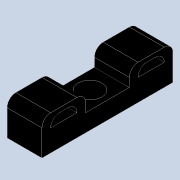
# Autodesk Inventor part: Wire Anchor
Saved by Autodesk Inventor 2022 (Build 260153000, 153)
## iProperties
Created: 2022-01-07
Part Number: Wire Anchor
Material: Generic
Document SubType Name: Modeling
Designer: Coy
Density: 1 g/cm^3
Appearance: Anodized - Black
Author: Coy
Autodesk Inventor part; units mm, degrees
ref_plane "YZ Plane" through (0, 0, 0) normal (1, 0, 0) x (0, 1, 0)
ref_plane "XZ Plane" through (0, 0, 0) normal (0, 1, 0) x (-1, 0, 0)
ref_plane "XY Plane" through (0, 0, 0) normal (0, 0, 1) x (1, 0, 0)
sketch "Sketch1" plane through (0, 0, 0) normal (1, 0, 0) x (0, 1, 0)
  line L0 (0, 0) -> (8, 0)
  line L1 (8, 0) -> (8, 30)
  line L2 (8, 30) -> (0, 30)
  line L3 (0, 30) -> (0, 0)
  line L4 (8, 10) -> (4, 10)
  line L5 (4, 10) -> (4, 20)
  line L6 (4, 20) -> (8, 20)
  line L7 (8, 20) -> (8, 10)
  dimension "d0" = 8
  dimension "d1" = 30
  dimension "d2" = 4
  dimension "d3" = 10
  dimension "d4" = 10
  constraints: 16 end point, 4 parallel, 2 horizontal, 2 perpendicular, 1 point on line
  measures "d0" distance of L2.end L1.end
  measures "d1" distance of L1.end L0.end
  measures "d2" distance of L5.end L6.end
  measures "d3" distance of L4.end L5.end
  measures "d4" distance between parallel lines of L0 L4
extrude "Extrusion1" add sketch "Sketch1" against normal blind 8 contours L3 L2 L1 L6 L5 L4 L0
sketch "Sketch2" plane through (0, 4, 20) normal (0, 1, 0) x (1, 0, 0)
  line L0 (0, 10) -> (0, 0) projected
  line L1 (0, 10) -> (-8, 10) projected
  line L2 (-8, 0) -> (-8, 10) projected
  line L3 (0, 0) -> (-8, 0) projected
  line L4 (-8, 0) -> (0, 10) construction
  line L5 (-8, 10) -> (0, 0) construction
  circle A0 centre (-4, 5) radius 2.75
  point P0 (0, 20)
  dimension "d7" = 5.5
  constraints: 4 end point, 1 centre point, 1 midpoint
  measures "d7" diameter of A0
extrude "Extrusion2" cut sketch "Sketch2" against normal up to next contours A0
sketch "Sketch3" plane through (0, 0, 0) normal (1, 0, 0) x (0, 0, -1)
  line L0 (0, 8) -> (-10, 8) projected
  line L1 (-10, 8) -> (-10, 4) projected
  line L2 (-10, 4) -> (-20, 4) projected
  line L3 (-20, 4) -> (-20, 8) projected
  line L4 (-20, 8) -> (-30, 8) projected
  line L5 (-30, 8) -> (-30, 0) projected
  line L6 (-30, 0) -> (0, 0) projected
  line L7 (0, 0) -> (0, 8) projected
  line L8 (-8, 7) -> (-2, 7)
  line L9 (-2, 7) -> (-2, 5)
  line L10 (-2, 5) -> (-8, 5)
  line L11 (-8, 5) -> (-8, 7)
  line L12 (-20, 4) -> (-10, 4) construction
  line L13 (-15, 4) -> (-15, 8) construction
  line L14 (-22, 7) -> (-28, 7)
  line L15 (-28, 7) -> (-28, 5)
  line L16 (-28, 5) -> (-22, 5)
  line L17 (-22, 5) -> (-22, 7)
  dimension "d10" = 6
  dimension "d11" = 2
  dimension "d12" = 10
  dimension "d13" = 2
  dimension "d14" = 4
  dimension "d15" = 1
  constraints: 18 end point, 4 symmetric about line, 2 parallel, 1 horizontal, 1 midpoint, 1 perpendicular, 1 vertical
  measures "d10" distance of L9.end L10.end
  measures "d11" distance of L8.end L9.end
  measures "d12" distance of L0.start L0.end
  measures "d13" distance between parallel lines of L1 L11
  measures "d14" distance of L0.end L1.end
  measures "d15" distance between parallel lines of L0 L8
extrude "Extrusion3" cut sketch "Sketch3" against normal up to next contours L8 L9 L10 L11 | L17 L16 L15 L14
fillet "Fillet1" radius 2 8 edges at (-4, 8, 10) (-4, 8, 20) (-4, 8, 30) (-4, 8, 0) (-4, 7, 28) (-4, 7, 22) (-4, 7, 8) (-4, 7, 2)
equation "\"d4\" = -0.5 * d3 + 0.5 * d1"
equation "\"d13\" = -0.5 * d10 + 0.5 * d12"
equation "\"d15\" = -0.5 * d11 + 0.5 * d14"
body "Solid1"
